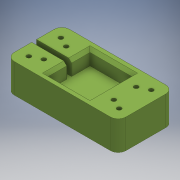
# Autodesk Inventor part: sujetador guia ejercedor presion
Saved by Autodesk Inventor 2018 (Build 220112000, 112)
## iProperties
Created: 2019-05-18
Part Number: sujetador guia ejercedor presion
Material: Generic
Document SubType Name: Modeling
Designer: JLVega003
Density: 1 g/cm^3
Appearance: Olive Green
Author: JLVega003
Autodesk Inventor part; units mm, degrees
ref_plane "YZ Plane" through (0, 0, 0) normal (1, 0, 0) x (0, 1, 0)
ref_plane "XZ Plane" through (0, 0, 0) normal (0, 1, 0) x (-1, 0, 0)
ref_plane "XY Plane" through (0, 0, 0) normal (0, 0, 1) x (1, 0, 0)
sketch "Sketch1" plane through (0, 0, 0) normal (0, 0, 1) x (1, 0, 0)
  line L0 (57.5, -28.5) -> (-57.5, -28.5)
  line L1 (-57.5, -28.5) -> (-57.5, 28.5)
  line L2 (-57.5, 28.5) -> (57.5, 28.5)
  line L3 (57.5, 28.5) -> (57.5, -28.5)
  line L4 (57.5, -28.5) -> (-57.5, 28.5) construction
  line L5 (-57.5, -28.5) -> (57.5, 28.5) construction
  line L6 (46.5, -16.5) -> (-46.5, -16.5) construction
  line L7 (-46.5, -16.5) -> (-46.5, 16.5) construction
  line L8 (-46.5, 16.5) -> (46.5, 16.5) construction
  line L9 (46.5, 16.5) -> (46.5, -16.5) construction
  line L10 (46.5, -16.5) -> (-46.5, 16.5) construction
  line L11 (-46.5, -16.5) -> (46.5, 16.5) construction
  line L12 (36, -11.5) -> (-36, -11.5) construction
  line L13 (-36, -11.5) -> (-36, 11.5) construction
  line L14 (-36, 11.5) -> (36, 11.5) construction
  line L15 (36, 11.5) -> (36, -11.5) construction
  line L16 (36, -11.5) -> (-36, 11.5) construction
  line L17 (-36, -11.5) -> (36, 11.5) construction
  circle A0 centre (-46.5, 16.5) radius 2.25
  circle A1 centre (-36, 11.5) radius 2.25
  circle A2 centre (-46.5, -16.5) radius 2.25
  circle A3 centre (-36, -11.5) radius 2.25
  circle A4 centre (46.5, -16.5) radius 2.25
  circle A5 centre (36, -11.5) radius 2.25
  circle A6 centre (36, 11.5) radius 2.25
  circle A7 centre (46.5, 16.5) radius 2.25
  point P0 (0, 0)
  dimension "d0" = 115
  dimension "d1" = 57
  dimension "d2" = 93
  dimension "d3" = 33
  dimension "d4" = 72
  dimension "d5" = 23
  dimension "d6" = 4.5
  constraints: 36 end point, 8 centre point, 8 coincident, 7 equal radius, 6 midpoint, 6 parallel, 3 horizontal, 3 perpendicular
  measures "d0" distance of L1.end L2.end
  measures "d1" distance of L0.end L1.end
  measures "d2" distance of L7.end L8.end
  measures "d3" distance of L6.end L7.end
  measures "d4" distance of L13.end L14.end
  measures "d5" distance of L12.end L13.end
  measures "d6" diameter of A0
extrude "Extrusion1" add sketch "Sketch1" along normal blind 30
sketch "Sketch2" plane through (0, 0, 0) normal (0, 0, -1) x (-1, 0, 0)
  circle A0 centre (-46.5, 16.5) radius 2.25 projected
  circle A1 centre (-36, 11.5) radius 2.25 projected
  circle A2 centre (-36, -11.5) radius 2.25 projected
  circle A3 centre (-46.5, -16.5) radius 2.25 projected
  circle A4 centre (36, -11.5) radius 2.25 projected
  circle A5 centre (46.5, -16.5) radius 2.25 projected
  circle A6 centre (36, 11.5) radius 2.25 projected
  circle A7 centre (46.5, 16.5) radius 2.25 projected
  line L0 (-57.5, -28.5) -> (57.5, -28.5) projected
  line L1 (57.5, -28.5) -> (57.5, 28.5) projected
  line L2 (57.5, 28.5) -> (-57.5, 28.5) projected
  line L3 (-57.5, 28.5) -> (-57.5, -28.5) projected
  circle A8 centre (-46.5, 16.5) radius 2.25 projected
  circle A9 centre (-46.5, 16.5) radius 6
  circle A10 centre (-46.5, -16.5) radius 2.25 projected
  circle A11 centre (-46.5, -16.5) radius 6
  circle A12 centre (46.5, -16.5) radius 6
  circle A13 centre (46.5, 16.5) radius 6
  point P0 (0, 0)
  dimension "d9" = 12
  constraints: 4 centre point, 4 coincident, 3 equal radius
  measures "d9" diameter of A9
extrude "Extrusion2" cut sketch "Sketch2" against normal blind 7 contours A9 | A11 | A12 | A13
sketch "Sketch6" plane through (0, 0, 30) normal (0, 0, 1) x (1, 0, 0)
  line L0 (21.5, -21.5) -> (-21.5, -21.5)
  line L1 (-21.5, -21.5) -> (-21.5, 21.5)
  line L2 (-21.5, 21.5) -> (21.5, 21.5)
  line L3 (21.5, 21.5) -> (21.5, -21.5)
  line L4 (21.5, -21.5) -> (-21.5, 21.5) construction
  line L5 (-21.5, -21.5) -> (21.5, 21.5) construction
  point P0 (0, 0)
  dimension "d27" = 43
  dimension "d28" = 43
  constraints: 12 end point, 2 midpoint, 2 parallel, 1 horizontal, 1 perpendicular
  measures "d27" distance of L1.end L2.end
  measures "d28" distance of L0.end L1.end
extrude "Extrusion5" cut sketch "Sketch6" against normal blind 15
sketch "Sketch7" plane through (0, 0, 0) normal (0, 1, 0) x (-1, 0, 0)
  line L0 (21.5, 30) -> (-21.5, 30) projected
  line L1 (21.5, 30) -> (21.5, 15) projected
  line L2 (21.5, 15) -> (-21.5, 15) projected
  line L3 (-21.5, 30) -> (-21.5, 15) projected
  line L4 (57.5, 0) -> (-57.5, 0) projected
  line L5 (57.5, 0) -> (57.5, 30) projected
  line L6 (-57.5, 30) -> (57.5, 30) projected
  line L7 (-57.5, 0) -> (-57.5, 30) projected
  line L8 (57.5, 30) -> (21.5, 30)
  line L9 (21.5, 30) -> (21.5, 15) projected
  line L10 (21.5, 15) -> (26.5, 15)
  line L11 (26.5, 15) -> (26.5, 25)
  line L12 (26.5, 25) -> (57.5, 25)
  line L13 (57.5, 30) -> (57.5, 25)
  line L14 (57.5, 0) -> (57.5, 30) projected
  point P0 (0, 0)
  dimension "d31" = 5
  dimension "d32" = 5
  constraints: 10 end point, 2 collinear, 2 perpendicular, 1 horizontal, 1 point on line
  measures "d31" distance between parallel lines of L12 L6
  measures "d32" distance between parallel lines of L1 L11
extrude "Extrusion6" cut sketch "Sketch7" along normal mid plane 5 contours L6 L5 L12 L11 L10 L1
chamfer "Chamfer2" distance 3 angle 45 6 edges at (-21.5, 12, 30) (0, 21.5, 30) (-21.5, -12, 30) (0, -21.5, 30) (21.5, 0, 30) (-26.5, 0, 25)
fillet "Fillet2" radius 8 4 edges at (-57.5, 28.5, 15) (-57.5, -28.5, 15) (57.5, -28.5, 15) (57.5, 28.5, 15)
body "Solid1"
